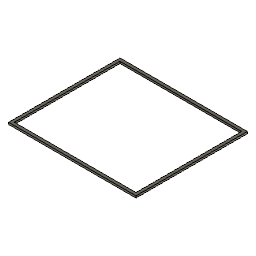
FanBoxGaskit (Autodesk Fusion 360 design; units mm, degrees)
Autodesk Fusion 360 part; units mm, degrees
sketch "Sketch1" plane through (0, 0, 0) normal (0, 0, 1) x (1, 0, 0)
  line L0 (0, 0) -> (128, 0)
  line L1 (128, 0) -> (128, 112)
  line L2 (128, 112) -> (0, 112)
  line L3 (0, 112) -> (0, 0)
  line L4 (3, 3) -> (125, 3)
  line L5 (125, 3) -> (125, 109)
  line L6 (125, 109) -> (3, 109)
  line L7 (3, 109) -> (3, 3)
  dimension "d1" = 128
  dimension "d2" = 112
  dimension "d3" = -3
  constraint horizontal L0
  constraint vertical L1
  constraint horizontal L2
  constraint vertical L3
  constraint coincident L0.start L3.end
  measures "d1" distance of L0.start L0.end
  measures "d2" distance of L0.start L2.end
extrude "Extrude1" add sketch "Sketch1" along normal blind 2
named bodies: "Gaskit"
